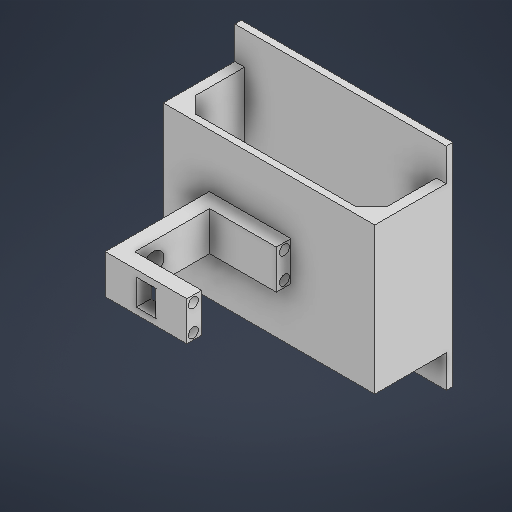
# Autodesk Inventor part: Base
Saved by Autodesk Inventor 2026 (Build 300175050, 175E)
## iProperties
Created: 2026-07-07
Part Number: Base
Material: 一般
Document SubType Name: Modeling
Designer: hanaj
Density: 1 g/cm^3
Appearance: 既定
Author: hanaj
Autodesk Inventor part; units mm, degrees
ref_plane "YZ Plane" through (0, 0, 0) normal (1, 0, 0) x (0, 1, 0)
ref_plane "XZ Plane" through (0, 0, 0) normal (0, 1, 0) x (-1, 0, 0)
ref_plane "XY Plane" through (0, 0, 0) normal (0, 0, 1) x (1, 0, 0)
sketch "スケッチ1" plane through (0, 0, 0) normal (0, 0, 1) x (1, 0, 0)
  line L0 (-32.5, 32.5) -> (32.5, 32.5)
  line L1 (32.5, 32.5) -> (32.5, -32.5)
  line L2 (32.5, -32.5) -> (-32.5, -32.5)
  line L3 (-32.5, -32.5) -> (-32.5, 32.5)
  line L4 (-32.5, 32.5) -> (32.5, -32.5) construction
  line L5 (32.5, 32.5) -> (-32.5, -32.5) construction
  line L6 (-27, 27) -> (27, 27) construction
  line L7 (27, 27) -> (27, -27) construction
  line L8 (27, -27) -> (-27, -27) construction
  line L9 (-27, -27) -> (-27, 27) construction
  line L10 (-27, 27) -> (27, -27) construction
  line L11 (27, 27) -> (-27, -27) construction
  point P0 (0, 0)
  dimension "d0" = 65
  dimension "d1" = 65
  dimension "d2" = 54
  dimension "d3" = 54
  constraints: 24 end point, 4 midpoint, 4 parallel, 2 horizontal, 2 perpendicular
  measures "d0" distance of L1.end L2.end
  measures "d1" distance of L0.end L1.end
  measures "d2" distance of L7.end L8.end
  measures "d3" distance of L6.end L7.end
extrude "押し出し1" add sketch "スケッチ1" along normal blind 2
sketch "スケッチ2" plane through (0, 0, 2) normal (0, 0, 1) x (1, 0, 0)
  line L0 (0, 54.4355) -> (0, -54.4355)
  line L1 (29.5, 22.5) -> (29.5, -22.5)
  line L2 (32.5, -32.5) -> (32.5, 32.5) projected
  line L3 (29.5, -22.5) -> (32.5, -22.5)
  line L4 (29.5, 22.5) -> (32.5, 22.5)
  line L5 (-36.7742, 0) -> (36.7742, 0)
  line L6 (-29.5, 22.5) -> (-29.5, -22.5)
  line L7 (-29.5, -22.5) -> (-32.5, -22.5)
  line L8 (-29.5, 22.5) -> (-32.5, 22.5)
  line L9 (-32.5, 32.5) -> (-32.5, -32.5) projected
  point P0 (0, 0)
  point P1 (32.5, 0)
  dimension "d7" = 22.5
  dimension "d8" = 45
  dimension "d9" = 3
  constraints: 16 end point, 4 symmetric about line, 3 midpoint, 2 perpendicular, 2 point on line, 2 vertical, 1 horizontal
  measures "d7" distance from line of point (32.5, 0) L4
  measures "d8" distance between parallel lines of L3 L4
  measures "d9" distance between parallel lines of L2 L1
extrude "押し出し2" add sketch "スケッチ2" along normal blind 20
sketch "スケッチ3" plane through (0, 0, 22) normal (0, 0, 1) x (1, 0, 0)
  line L0 (-32.5, -22.5) -> (-29.5, -22.5) projected
  line L1 (-29.5, -22.5) -> (-29.5, 22.5) projected
  line L2 (-29.5, 22.5) -> (-32.5, 22.5) projected
  line L3 (-32.5, 22.5) -> (-32.5, -22.5) projected
  line L4 (29.5, -22.5) -> (32.5, -22.5) projected
  line L5 (32.5, -22.5) -> (32.5, 22.5) projected
  line L6 (32.5, 22.5) -> (29.5, 22.5) projected
  line L7 (29.5, 22.5) -> (29.5, -22.5) projected
  line L8 (32.5, -22.5) -> (-32.5, -22.5)
  line L9 (-32.5, -22.5) -> (-32.5, 22.5)
  line L10 (-32.5, 22.5) -> (32.5, 22.5)
  line L11 (32.5, 22.5) -> (32.5, -22.5)
  point P0 (0, 0)
  constraints: 8 end point, 2 parallel, 1 horizontal, 1 perpendicular
extrude "押し出し3" add sketch "スケッチ3" along normal blind 2
sketch "スケッチ4" plane through (0, 0, 24) normal (0, 0, 1) x (1, 0, 0)
  line L0 (13.75, -6) -> (-13.75, -6)
  line L1 (-13.75, -6) -> (-13.75, 6)
  line L2 (-13.75, 6) -> (13.75, 6)
  line L3 (13.75, 6) -> (13.75, -6)
  line L4 (13.75, -6) -> (-13.75, 6) construction
  line L5 (-13.75, -6) -> (13.75, 6) construction
  line L6 (-13.75, -6) -> (6.75, -6)
  line L7 (6.75, -6) -> (6.75, 6)
  line L8 (6.75, 6) -> (-13.75, 6)
  line L9 (-13.75, 6) -> (-13.75, -6)
  point P0 (0, 0)
  point P1 (6.75, -6)
  dimension "d14" = 27.5
  dimension "d15" = 12
  dimension "d16" = 7
  constraints: 20 end point, 4 parallel, 2 horizontal, 2 midpoint, 2 perpendicular, 1 point on line
  measures "d14" distance of L1.end L2.end
  measures "d15" distance of L0.end L1.end
  measures "d16" distance between parallel lines of L7 L3
extrude "押し出し4" add sketch "スケッチ4" along normal blind 4.5 contours L0 L1 L2 L7
sketch "スケッチ5" plane through (0, 0, 24) normal (0, 0, 1) x (1, 0, 0)
  line L0 (-13.75, -6) -> (-13.75, 6) projected
  line L1 (-13.75, -6) -> (-19.35, -6)
  line L2 (-19.35, -6) -> (-19.35, 6)
  line L3 (-19.35, 6) -> (-13.75, 6)
  line L4 (-13.75, 6) -> (-13.75, -6)
  line L5 (6.75, 6) -> (-13.75, 6) projected
  point P0 (0, 0)
  dimension "d19" = 5.6
  constraints: 8 end point, 2 parallel, 1 collinear, 1 horizontal, 1 perpendicular
  measures "d19" distance between parallel lines of L2 L0
extrude "押し出し5" add sketch "スケッチ5" along normal blind 32
sketch "スケッチ6" plane through (-13.75, -6, 28.5) normal (1, 0, 0) x (0, 0, -1)
  line L0 (0, 12) -> (0, 0) projected
  line L1 (0, 12) -> (-27.5, 12) projected
  line L2 (-27.5, 0) -> (-27.5, 12) projected
  line L3 (0, 0) -> (-27.5, 0) projected
  line L4 (-23, 0) -> (-23, 12)
  point P0 (28.5, 6)
  dimension "d22" = 4.5
  constraints: 2 end point, 2 point on line, 1 vertical
  measures "d22" distance between parallel lines of L4 L2
extrude "押し出し6" add sketch "スケッチ6" along normal blind 20.5 contours L4 L3 L2 L1
sketch "スケッチ7" plane through (-19.35, -6, 24) normal (-1, 0, 0) x (0, 0, 1)
  line L0 (32, 12) -> (32, 0) construction
  line L1 (32, 6) -> (0, 6) construction
  line L2 (0, 28.5) -> (0, -16.5) construction
  point P0 (-24, 6)
  point P1 (21.79, 6)
  dimension "d25" = 10.21
  constraints: 2 end point, 2 midpoint, 1 point on line
  measures "d25" distance from line of point (21.79, 6) L0
hole "穴1" at (-19.35, 0, 45.79) direction (1, 0, 0) diameter 6.4 depth 6.3
sketch "スケッチ8" plane through (-19.35, -6, 24) normal (-1, 0, 0) x (0, 0, 1)
  circle A0 centre (21.79, 6) radius 3.2 projected
  line L0 (0, 0) -> (0, 12) projected
  line L1 (0, 0) -> (32, 0) projected
  line L2 (32, 12) -> (32, 0) projected
  line L3 (0, 12) -> (32, 12) projected
  point P0 (-24, 6)
extrude "押し出し7" cut sketch "スケッチ8" against normal blind 1
sketch "スケッチ9" plane through (6.75, -6, 24) normal (1, 0, 0) x (0, 0, -1)
  circle A0 centre (-21.79, 6) radius 3.2 projected
  line L0 (-58.0849, 6) -> (14.5049, 6)
  line L1 (0, -16.5) -> (0, 28.5) projected
  line L2 (-16, -14.4154) -> (-16, 26.4154)
  line L3 (-32, 12) -> (-32, 0) projected
  point P0 (24, 6)
  point P1 (-2, 2)
  point P2 (-2, 10)
  point P3 (-16, 6)
  point P4 (-30, 2)
  point P5 (-30, 10)
  dimension "d35" = 8
  dimension "d36" = 2
  dimension "d37" = 16
  constraints: 4 end point, 3 symmetric about line, 2 midpoint, 1 horizontal, 1 point on line, 1 vertical
  measures "d35" diameter of point (-2, 2) L0
  measures "d36" distance from line of L1 point (-2, 2)
  measures "d37" distance between parallel lines of L2 L3
hole "穴2" at (6.75, -4, 26) at (6.75, 4, 26) at (6.75, -4, 54) at (6.75, 4, 54) direction (-1, 0, 0) diameter 3 depth 3
sketch "スケッチ10" plane through (0, 0, 2) normal (0, 0, 1) x (1, 0, 0)
  line L0 (24.25, -0.35) -> (-24.25, -0.35)
  line L1 (-24.25, -0.35) -> (-24.25, 28.35)
  line L2 (-24.25, 28.35) -> (24.25, 28.35)
  line L3 (24.25, 28.35) -> (24.25, -0.35)
  line L4 (24.25, -0.35) -> (-24.25, 28.35) construction
  line L5 (-24.25, -0.35) -> (24.25, 28.35) construction
  line L6 (32.5, 22.5) -> (32.5, 32.5) projected
  line L7 (32.5, 32.5) -> (-32.5, 32.5) projected
  circle A0 centre (24.25, -0.35) radius 3
  circle A1 centre (24.25, 28.35) radius 3
  circle A2 centre (-24.25, 28.35) radius 3
  circle A3 centre (-24.25, -0.35) radius 3
  point P0 (0, 0)
  point P1 (0, 14)
  point P2 (32.5, 27.5)
  dimension "d45" = 48.5
  dimension "d46" = 28.7
  dimension "d47" = 32.5
  dimension "d48" = 18.5
  dimension "d56" = 6
  dimension "d57" = 6
  dimension "d58" = 6
  dimension "d59" = 6
  constraints: 12 end point, 8 coincident, 4 centre point, 3 midpoint, 2 parallel, 1 horizontal, 1 perpendicular
  measures "d45" distance of L1.end L2.end
  measures "d46" distance of L0.end L1.end
  measures "d47" horizontal distance of point (0, 14) point (32.5, 27.5)
  measures "d48" distance from line of L7 point (0, 14)
  measures "d56" diameter of A0
  measures "d57" diameter of A1
  measures "d58" diameter of A2
  measures "d59" diameter of A3
extrude "押し出し8" [suppressed]
sketch "スケッチ11" plane through (0, 0, 0) normal (0, 0, -1) x (-1, 0, 0)
  circle A0 centre (-24.25, 28.35) radius 3 projected
  circle A1 centre (-24.25, -0.35) radius 3 projected
  circle A2 centre (24.25, -0.35) radius 3 projected
  circle A3 centre (24.25, 28.35) radius 3 projected
  point P0 (0, 0)
  point P1 (-18.5, 30)
  constraints: 1 other
hole "穴4" [suppressed]
chamfer "面取り1" distance 5 angle 45 2 edges at (29.5, 0, 22) (-29.5, 0, 22)
fillet "フィレット1" [suppressed]
sketch "スケッチ12" plane through (0, 0, 56) normal (0, 0, 1) x (1, 0, 0)
  line L0 (-2.75, -4) -> (-8.75, -4)
  line L1 (-8.75, -4) -> (-8.75, 4)
  line L2 (-8.75, 4) -> (-2.75, 4)
  line L3 (-2.75, 4) -> (-2.75, -4)
  line L4 (-2.75, -4) -> (-8.75, 4) construction
  line L5 (-8.75, -4) -> (-2.75, 4) construction
  line L6 (-13.75, 6) -> (-13.75, -6) projected
  line L7 (-18.35, -6) -> (6.75, -6) projected
  point P0 (0, 0)
  point P1 (-5.75, 0)
  dimension "d73" = 6
  dimension "d74" = 8
  dimension "d75" = 5
  dimension "d76" = 6
  constraints: 12 end point, 2 midpoint, 2 parallel, 1 horizontal, 1 perpendicular
  measures "d73" distance of L1.end L2.end
  measures "d74" distance of L0.end L1.end
  measures "d75" distance between parallel lines of L6 L1
  measures "d76" distance from line of L7 point (-5.75, 0)
extrude "押し出し9" cut sketch "スケッチ12" against normal blind 6.75
